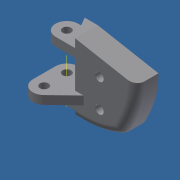
# Autodesk Inventor part: FingerTipp
Saved by Autodesk Inventor 2014 SP2 (Build 180246200, 246)
## iProperties
Created: 2014-12-28
Part Number: FingerTipp
Material: Generisch
Document SubType Name: Modeling
Designer: 4ndreas
Density: 1 g/cm^3
Appearance: Vorgabe
Mass: 3.82161 g
Surface Area: 22.4726 cm^2
Volume: 3.82161 cm^3
Author: 4ndreas
Autodesk Inventor part; units mm, degrees
ref_plane "YZ Plane" through (0, 0, 0) normal (1, 0, 0) x (0, 1, 0)
ref_plane "XZ Plane" through (0, 0, 0) normal (0, 1, 0) x (-1, 0, 0)
ref_plane "XY Plane" through (0, 0, 0) normal (0, 0, 1) x (1, 0, 0)
sketch "Skizze1" plane through (0, 0, 0) normal (0, 0, 1) x (1, 0, 0)
  circle A0 centre (0, 0) radius 4
  line L0 (2.3094, 4) -> (9.9282, 4)
  line L1 (9.9282, 4) -> (9.9282, -4)
  line L2 (9.9282, -4) -> (6.9282, -4)
  line L3 (6.9282, -4) -> (2.3094, 4)
  line L4 (0, -4) -> (6.9282, -4)
  line L5 (2.3094, 4) -> (0, 4)
  dimension "d0" = 8
  dimension "d2" = 60
  dimension "d10" = 3
  constraints: 12 end point, 4 tangent, 2 collinear, 2 perpendicular, 2 point on circle, 1 centre point, 1 coincident, 1 horizontal
  measures "d0" diameter of A0
  measures "d2" angle of L3 L0
  measures "d10" distance from line of L2.end L1
extrude "Extrusion1" add sketch "Skizze1" along normal blind 3
extrude "Extrusion2" add sketch "Skizze1" against normal blind 3 contours L3 L0 L1 L2
sketch "Skizze2" plane through (0, 0, 3) normal (0, 0, 1) x (1, 0, 0)
  line L0 (2.3094, 4) -> (9.9282, 4) projected
  line L1 (9.9282, 4) -> (9.9282, -4) projected
  line L2 (9.9282, -4) -> (6.9282, -4) projected
  line L3 (6.9282, -4) -> (2.3094, 4) projected
  line L4 (6.9282, -4) -> (9.9282, -4)
  line L5 (9.9282, -4) -> (9.9282, 4)
  line L6 (9.9282, 4) -> (6.9282, 4)
  line L7 (6.9282, 4) -> (6.9282, -4)
  constraints: 8 end point, 2 parallel, 1 horizontal, 1 perpendicular
extrude "Extrusion3" add sketch "Skizze2" along normal blind 6.5 contours L0 L1 L2 L7
mirror "Spiegeln1" about plane through (8.4282, 0, 9.5) normal (0, 0, 1)
sketch "Skizze4" plane through (0, 0, 3) normal (0, 0, 1) x (1, 0, 0)
  line L0 (6.9282, -4) -> (6.9282, 4) projected
  line L1 (6.9282, 4) -> (0, 4) projected
  arc A0 (0, 4) -> (0, -4) centre (0, 0) ccw projected
  line L2 (0, -4) -> (6.9282, -4) projected
  line L3 (2.3094, 4) -> (9.9282, 4) projected
  line L4 (9.9282, 4) -> (9.9282, -4) projected
  line L5 (9.9282, -4) -> (6.9282, -4) projected
  line L6 (6.9282, -4) -> (2.3094, 4) projected
  line L7 (-4, 0) -> (-4, -8)
  line L8 (0, 0) -> (0, -8) construction
  line L9 (9.9282, -4) -> (2.773, -10.8828)
  arc A1 (-4, -8) -> (2.773, -10.8828) centre (0, -8) ccw
  arc A2 (0, 4) -> (-4, 0) centre (0, 0) ccw
  line L10 (0, 4) -> (9.9282, 4)
  line L11 (9.9282, -4) -> (9.9282, 4)
  dimension "d18" = 8
  constraints: 10 end point, 5 point on circle, 2 centre point, 2 coincident, 2 parallel, 2 tangent, 1 equal radius, 1 perpendicular
  measures "d18" distance of L8.start L8.end
extrude "Extrusion4" [suppressed]
extrude "Extrusion5" add sketch "Skizze4" along normal blind 3
sketch "Skizze5" plane through (0, 0, -3) normal (0, 0, -1) x (-1, 0, 0)
  line L0 (-2.3094, 4) -> (-6.9282, -4) projected
  line L1 (0, -4) -> (-6.9282, -4) projected
  arc A0 (0, -4) -> (0, 4) centre (0, 0) ccw projected
  line L2 (-2.3094, 4) -> (0, 4) projected
  line L3 (0, -4) -> (-9.9282, -4) projected
  line L4 (-2.773, -10.8828) -> (-9.9282, -4) projected
  arc A1 (-2.773, -10.8828) -> (4, -8) centre (0, -8) ccw projected
  line L5 (4, 0) -> (4, -8) projected
  arc A2 (0, -4) -> (4, 0) centre (0, 0) ccw projected
hole "Bohrung2" at (0, 0, -3) at (0, -8, -3) direction (0, 0, 1) diameter 3 end through all
sketch "Skizze7" plane through (0, 4, 0) normal (0, 1, 0) x (1, 0, 0)
  line L0 (9.9282, 3) -> (9.9282, -22) projected
  line L1 (2.3094, 3) -> (9.9282, 3) projected
  line L2 (0, 0) -> (0, -6) projected
  line L3 (6.9282, -6) -> (0, -6) projected
  line L4 (9.9282, 3) -> (16.8306, 3) construction
  line L5 (16.8306, 3) -> (23.047, 0) construction
  spline S0 degree 2 poles (9.9282, 3) (16.8306, 3) (23.047, 0) knots 1 1 1 2 2 2
  arc A0 (24.9282, -9.5) -> (23.047, 0) centre (0, -9.5) ccw
  line L6 (9.9282, -9.5) -> (32.3299, -9.5) construction
  line L7 (23.047, 0) -> (2.3094, 0) construction
  line L8 (9.9282, -22) -> (16.8306, -22) construction
  line L9 (16.8306, -22) -> (23.047, -19) construction
  spline S1 degree 2 poles (9.9282, -22) (16.8306, -22) (23.047, -19) knots 1 1 1 2 2 2
  arc A1 (23.047, -19) -> (24.9282, -9.5) centre (0, -9.5) ccw
  dimension "d30" = 15
  constraints: 4 end point, 4 point on circle, 3 point on line, 2 centre point, 2 symmetric about line, 1 collinear, 1 equal length, 1 midpoint, 1 parallel, 1 perpendicular, 7 other
  measures "d30" distance from line of A0.start L0
extrude "Extrusion6" add sketch "Skizze7" against normal up to surface (8 mm away)
sketch "Skizze8" plane through (0, -4, 16) normal (0, -1, 0) x (1, 0, 0)
  arc A0 (19.9211, -13.9956) -> (20.4401, 0.0137) centre (6.9282, -6.5) ccw
  line L0 (9.9282, -13) -> (9.9282, -10)
  line L1 (0, -16) -> (6.9282, -16)
  line L2 (6.9282, -6.5) -> (21.9282, -6.5)
  line L3 (9.9282, -11.5) -> (21.0703, -11.5)
  arc A1 (23.047, -16) -> (23.047, 3) centre (0, -6.5) ccw projected
  line L4 (6.9282, -10) -> (6.9282, 0) projected
  point P0 (15.4993, -1.5)
  point P1 (15.4993, -11.5)
  dimension "d55" = 3
  constraints: 8 end point, 4 point on circle, 2 midpoint, 2 parallel, 2 point on line, 1 centre point, 1 coincident, 1 symmetric about line
hole "Bohrung3" at (15.4993, -4, 14.5) at (15.4993, -4, 4.5) direction (0, 1, 0) diameter 3 end through all
chamfer "Fase3" distance 1 angle 45 2 edges at (15.4993, 4, 6) (15.4993, 4, 16)
sketch "Skizze12" plane through (0, -4, 0) normal (0, -1, 0) x (1, 0, 0)
  spline S0 degree 2 poles (9.9282, 22) (16.8306, 22) (23.047, 19) knots 0 0 0 1 1 1 projected
  line L0 (9.9282, 22) -> (6.9282, 22) projected
  line L1 (6.9282, 22) -> (23.047, 19)
  constraints: 2 end point, 1 other
extrude "Extrusion10" cut sketch "Skizze12" against normal through all
sketch "Skizze13" plane through (0, -4, 0) normal (0, -1, 0) x (1, 0, 0)
  line L0 (23.047, 19) -> (6.9282, 22) projected
  line L1 (6.9282, 6) -> (6.9282, 16) projected
  arc A0 (23.047, 0) -> (23.047, 19) centre (0, 9.5) ccw projected
  line L2 (23.047, 19) -> (28.3554, 18.012)
  line L3 (23.047, 0) -> (28.3554, 9.2178) construction
  line L4 (28.3554, 9.2178) -> (28.3554, 18.012) construction
  spline S0 degree 2 poles (23.047, 0) (28.3554, 9.2178) (28.3554, 18.012) knots 1 1 1 2 2 2
  constraints: 2 end point, 1 collinear, 1 parallel, 3 other
extrude "Extrusion11" add sketch "Skizze13" against normal up to surface (8 mm away)
fillet "Rundung2" radius 3 4 edges at (23.047, 0, 0) (27.0283, -4, 9.1119) (8.4282, -4, -3) (16.6591, -4, -2.25)
equation "\"d0\" = Finger_diameter"
equation "\"d10\" = FingerWall"
equation "\"d4\" = FingerWall"
equation "\"d6\" = FingerWall"
equation "\"d8\" = -1.5 * FingerWall + 0.5 * Finger_width"
equation "\"d18\" = Finger_diameter"
equation "\"d23\" = bearingHole"
equation "\"FingerLaenge_B\" = 25"
equation "\"Hebel_B\" = 25"
equation "\"Finger_width\" = 22"
equation "\"Finger_diameter\" = 8"
equation "\"FingerWall\" = 3"
equation "\"Hebel_basis_2\" = 15"
equation "\"Join_width\" = 3"
equation "\"bearingHole\" = 3"
equation "\"bearingWall\" = 4"
equation "\"support_D\" = 0.25"
